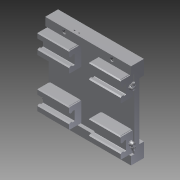
# Autodesk Inventor part: GL20NL-typeExNY Table
Saved by Autodesk Inventor 2011 SP1 (Build 150282100, 282)
## iProperties
Created: 2013-11-12
Part Number: GL20NL-typeExNY Table
Catalog Web Link: www.cadenas.de
Description: Type GL-N-Y - Table2-
Vendor: THK
Document SubType Name: Modeling
Designer: PARTuser1
Manufacturer: THK
Density: 1 g/cm^3
Category: PARTsolutions
Company: THK
Title: GL20NL-typeExNY Table
Author: Cadenas PARTsolutions
PSOL_IDENT_0: {$CADENAS_DATA\23d-libs\thk\actuator\type_gl_n\type_gl_n_f_na_s20.prj},199 {VTYP=3D},{NB=GL20NL-type
PSOL_IDENT_1: ExNY Table},{LINA=GL20NL-typeExNY Table},{NN=Type GL-N-Y - Table2},{DATE=01.03.2011 00:58:01},{GEOMD
PSOL_IDENT_2: ATE=14.11.2007 13:42:00},{VERSION=},{LINEID=60},{LINESUBID=-1},{WBVAR=S}  {NB=GL20NL-typeExNY Table}
PSOL_IDENT_3: ,{LINA=GL20NL-typeExNY Table},{KT=DUMMY},{IDNR=},{MN=GL20N},{TT=L-type},{TL=180},{B=55},{C=100},{D=2
PSOL_IDENT_4: 7},{RF=5.000},{RF2=2.750},{L1=62.000},{L2=66.500},{DS=Ex},{VER=2},{S=N},{LM=SW}
CNS_NN: Type GL-N-Y - Table2
CNS_NB: GL20NL-typeExNY Table
CNS_NBSYN: $MN.$TT.$DS.$S.Y Table
CNS_LINA: GL20NL-typeExNY Table
CNS_MN: GL20N
CNS_TT: L-type
CNS_TL: 180
CNS_B: 55
CNS_C: 100
CNS_D: 27
CNS_RF: 5.000
CNS_RF2: 2.750
CNS_L1: 62.000
CNS_L2: 66.500
CNS_DS: Ex
CNS_VER: 2
CNS_S: N:None
CNS_LM: SW
SUPPLIER: THK
ARTICLENO: GL20NL-typeExNY Table
BOMINFO: GL20NL-typeExNY Table
CREATOR: CADENAS GmbH
Autodesk Inventor part; units mm, degrees
sketch "Sketch_2" plane through (0, 0, 0) normal (1, 0, 0) x (0, 1, 0)
  line L0 (19, 90) -> (19, 73)
  line L1 (19, 73) -> (26, 73)
  line L2 (26, 73) -> (26, -73)
  line L3 (26, -73) -> (19, -73)
  line L4 (19, -73) -> (19, -90)
  line L5 (19, -90) -> (46, -90)
  line L6 (46, -90) -> (46, -60)
  line L7 (46, -60) -> (36.5, -60)
  line L8 (36.5, -60) -> (36.5, 60)
  line L9 (36.5, 60) -> (46, 60)
  line L10 (46, 60) -> (46, 90)
  line L11 (46, 90) -> (19, 90)
  constraints: 24 end point
extrude "Extrusion1" add sketch "Sketch_2" along normal mid plane 180
sketch "Sketch_3" plane through (85, 0, 0) normal (1, 0, 0) x (0, 0, -1)
  line L0 (29.75, 25) -> (29.75, 1.8)
  line L1 (29.75, 1.8) -> (30.5, 1.05)
  line L2 (30.5, 1.05) -> (30.5, 24.6)
  line L3 (30.5, 24.6) -> (31.5, 25.6)
  line L4 (31.5, 25.6) -> (45.55, 25.6)
  line L5 (45.55, 25.6) -> (45.25, 26)
  line L6 (45.25, 26) -> (30.75, 26)
  line L7 (30.75, 26) -> (29.75, 25)
  constraints: 16 end point
extrude "Extrusion2" add sketch "Sketch_3" against normal blind 62
sketch "Sketch_4" plane through (85, 0, 0) normal (1, 0, 0) x (0, 0, -1)
  line L0 (56.45, 25.6) -> (70.5, 25.6)
  line L1 (70.5, 25.6) -> (71.5, 24.6)
  line L2 (71.5, 24.6) -> (71.5, 1.05)
  line L3 (71.5, 1.05) -> (72.25, 1.8)
  line L4 (72.25, 1.8) -> (72.25, 25)
  line L5 (72.25, 25) -> (71.25, 26)
  line L6 (71.25, 26) -> (56.75, 26)
  line L7 (56.75, 26) -> (56.45, 25.6)
  constraints: 16 end point
extrude "Extrusion3" add sketch "Sketch_4" against normal blind 62
sketch "Sketch_5" plane through (87.25, 0, 0) normal (1, 0, 0) x (0, 0, -1)
  line L0 (30.5, 24.6) -> (30.5, 1)
  line L1 (30.5, 1) -> (31.5, 0)
  line L2 (31.5, 0) -> (40.7, 0)
  line L3 (40.7, 0) -> (42.7, 2)
  line L4 (42.7, 2) -> (42.7, 5.5)
  line L5 (42.7, 5.5) -> (40.7, 7.5)
  line L6 (40.7, 7.5) -> (40.7, 10.72)
  line L7 (40.7, 10.72) -> (41.48, 11.5)
  line L8 (41.48, 11.5) -> (60.52, 11.5)
  line L9 (60.52, 11.5) -> (61.3, 10.72)
  line L10 (61.3, 10.72) -> (61.3, 7.5)
  line L11 (61.3, 7.5) -> (59.3, 5.5)
  line L12 (59.3, 5.5) -> (59.3, 2)
  line L13 (59.3, 2) -> (61.3, 0)
  line L14 (61.3, 0) -> (70.5, 0)
  line L15 (70.5, 0) -> (71.5, 1)
  line L16 (71.5, 1) -> (71.5, 24.6)
  line L17 (71.5, 24.6) -> (70.5, 25.6)
  line L18 (70.5, 25.6) -> (31.5, 25.6)
  line L19 (31.5, 25.6) -> (30.5, 24.6)
  constraints: 40 end point
extrude "Extrusion4" add sketch "Sketch_5" against normal blind 66.5
sketch "Sketch_6" plane through (85, 0, 0) normal (1, 0, 0) x (0, 0, -1)
  line L0 (-72.25, 25) -> (-72.25, 1.8)
  line L1 (-72.25, 1.8) -> (-71.5, 1.05)
  line L2 (-71.5, 1.05) -> (-71.5, 24.6)
  line L3 (-71.5, 24.6) -> (-70.5, 25.6)
  line L4 (-70.5, 25.6) -> (-56.45, 25.6)
  line L5 (-56.45, 25.6) -> (-56.75, 26)
  line L6 (-56.75, 26) -> (-71.25, 26)
  line L7 (-71.25, 26) -> (-72.25, 25)
  constraints: 16 end point
extrude "Extrusion5" add sketch "Sketch_6" against normal blind 62
sketch "Sketch_7" plane through (85, 0, 0) normal (1, 0, 0) x (0, 0, -1)
  line L0 (-45.55, 25.6) -> (-31.5, 25.6)
  line L1 (-31.5, 25.6) -> (-30.5, 24.6)
  line L2 (-30.5, 24.6) -> (-30.5, 1.05)
  line L3 (-30.5, 1.05) -> (-29.75, 1.8)
  line L4 (-29.75, 1.8) -> (-29.75, 25)
  line L5 (-29.75, 25) -> (-30.75, 26)
  line L6 (-30.75, 26) -> (-45.25, 26)
  line L7 (-45.25, 26) -> (-45.55, 25.6)
  constraints: 16 end point
extrude "Extrusion6" add sketch "Sketch_7" against normal blind 62
sketch "Sketch_8" plane through (87.25, 0, 0) normal (1, 0, 0) x (0, 0, -1)
  line L0 (-71.5, 24.6) -> (-71.5, 1)
  line L1 (-71.5, 1) -> (-70.5, 0)
  line L2 (-70.5, 0) -> (-61.3, 0)
  line L3 (-61.3, 0) -> (-59.3, 2)
  line L4 (-59.3, 2) -> (-59.3, 5.5)
  line L5 (-59.3, 5.5) -> (-61.3, 7.5)
  line L6 (-61.3, 7.5) -> (-61.3, 10.72)
  line L7 (-61.3, 10.72) -> (-60.52, 11.5)
  line L8 (-60.52, 11.5) -> (-41.48, 11.5)
  line L9 (-41.48, 11.5) -> (-40.7, 10.72)
  line L10 (-40.7, 10.72) -> (-40.7, 7.5)
  line L11 (-40.7, 7.5) -> (-42.7, 5.5)
  line L12 (-42.7, 5.5) -> (-42.7, 2)
  line L13 (-42.7, 2) -> (-40.7, 0)
  line L14 (-40.7, 0) -> (-31.5, 0)
  line L15 (-31.5, 0) -> (-30.5, 1)
  line L16 (-30.5, 1) -> (-30.5, 24.6)
  line L17 (-30.5, 24.6) -> (-31.5, 25.6)
  line L18 (-31.5, 25.6) -> (-70.5, 25.6)
  line L19 (-70.5, 25.6) -> (-71.5, 24.6)
  constraints: 40 end point
extrude "Extrusion7" add sketch "Sketch_8" against normal blind 66.5
sketch "Sketch_9" plane through (-85, 0, 0) normal (1, 0, 0) x (0, 0, -1)
  line L0 (29.75, 25) -> (29.75, 1.8)
  line L1 (29.75, 1.8) -> (30.5, 1.05)
  line L2 (30.5, 1.05) -> (30.5, 24.6)
  line L3 (30.5, 24.6) -> (31.5, 25.6)
  line L4 (31.5, 25.6) -> (45.55, 25.6)
  line L5 (45.55, 25.6) -> (45.25, 26)
  line L6 (45.25, 26) -> (30.75, 26)
  line L7 (30.75, 26) -> (29.75, 25)
  constraints: 16 end point
extrude "Extrusion8" add sketch "Sketch_9" along normal blind 62
sketch "Sketch_10" plane through (-85, 0, 0) normal (1, 0, 0) x (0, 0, -1)
  line L0 (56.45, 25.6) -> (70.5, 25.6)
  line L1 (70.5, 25.6) -> (71.5, 24.6)
  line L2 (71.5, 24.6) -> (71.5, 1.05)
  line L3 (71.5, 1.05) -> (72.25, 1.8)
  line L4 (72.25, 1.8) -> (72.25, 25)
  line L5 (72.25, 25) -> (71.25, 26)
  line L6 (71.25, 26) -> (56.75, 26)
  line L7 (56.75, 26) -> (56.45, 25.6)
  constraints: 16 end point
extrude "Extrusion9" add sketch "Sketch_10" along normal blind 62
sketch "Sketch_11" plane through (-87.25, 0, 0) normal (1, 0, 0) x (0, 0, -1)
  line L0 (30.5, 24.6) -> (30.5, 1)
  line L1 (30.5, 1) -> (31.5, 0)
  line L2 (31.5, 0) -> (40.7, 0)
  line L3 (40.7, 0) -> (42.7, 2)
  line L4 (42.7, 2) -> (42.7, 5.5)
  line L5 (42.7, 5.5) -> (40.7, 7.5)
  line L6 (40.7, 7.5) -> (40.7, 10.72)
  line L7 (40.7, 10.72) -> (41.48, 11.5)
  line L8 (41.48, 11.5) -> (60.52, 11.5)
  line L9 (60.52, 11.5) -> (61.3, 10.72)
  line L10 (61.3, 10.72) -> (61.3, 7.5)
  line L11 (61.3, 7.5) -> (59.3, 5.5)
  line L12 (59.3, 5.5) -> (59.3, 2)
  line L13 (59.3, 2) -> (61.3, 0)
  line L14 (61.3, 0) -> (70.5, 0)
  line L15 (70.5, 0) -> (71.5, 1)
  line L16 (71.5, 1) -> (71.5, 24.6)
  line L17 (71.5, 24.6) -> (70.5, 25.6)
  line L18 (70.5, 25.6) -> (31.5, 25.6)
  line L19 (31.5, 25.6) -> (30.5, 24.6)
  constraints: 40 end point
extrude "Extrusion10" add sketch "Sketch_11" along normal blind 66.5
sketch "Sketch_12" plane through (-85, 0, 0) normal (1, 0, 0) x (0, 0, -1)
  line L0 (-72.25, 25) -> (-72.25, 1.8)
  line L1 (-72.25, 1.8) -> (-71.5, 1.05)
  line L2 (-71.5, 1.05) -> (-71.5, 24.6)
  line L3 (-71.5, 24.6) -> (-70.5, 25.6)
  line L4 (-70.5, 25.6) -> (-56.45, 25.6)
  line L5 (-56.45, 25.6) -> (-56.75, 26)
  line L6 (-56.75, 26) -> (-71.25, 26)
  line L7 (-71.25, 26) -> (-72.25, 25)
  constraints: 16 end point
extrude "Extrusion11" add sketch "Sketch_12" along normal blind 62
sketch "Sketch_13" plane through (-85, 0, 0) normal (1, 0, 0) x (0, 0, -1)
  line L0 (-45.55, 25.6) -> (-31.5, 25.6)
  line L1 (-31.5, 25.6) -> (-30.5, 24.6)
  line L2 (-30.5, 24.6) -> (-30.5, 1.05)
  line L3 (-30.5, 1.05) -> (-29.75, 1.8)
  line L4 (-29.75, 1.8) -> (-29.75, 25)
  line L5 (-29.75, 25) -> (-30.75, 26)
  line L6 (-30.75, 26) -> (-45.25, 26)
  line L7 (-45.25, 26) -> (-45.55, 25.6)
  constraints: 16 end point
extrude "Extrusion12" add sketch "Sketch_13" along normal blind 62
sketch "Sketch_14" plane through (-87.25, 0, 0) normal (1, 0, 0) x (0, 0, -1)
  line L0 (-71.5, 24.6) -> (-71.5, 1)
  line L1 (-71.5, 1) -> (-70.5, 0)
  line L2 (-70.5, 0) -> (-61.3, 0)
  line L3 (-61.3, 0) -> (-59.3, 2)
  line L4 (-59.3, 2) -> (-59.3, 5.5)
  line L5 (-59.3, 5.5) -> (-61.3, 7.5)
  line L6 (-61.3, 7.5) -> (-61.3, 10.72)
  line L7 (-61.3, 10.72) -> (-60.52, 11.5)
  line L8 (-60.52, 11.5) -> (-41.48, 11.5)
  line L9 (-41.48, 11.5) -> (-40.7, 10.72)
  line L10 (-40.7, 10.72) -> (-40.7, 7.5)
  line L11 (-40.7, 7.5) -> (-42.7, 5.5)
  line L12 (-42.7, 5.5) -> (-42.7, 2)
  line L13 (-42.7, 2) -> (-40.7, 0)
  line L14 (-40.7, 0) -> (-31.5, 0)
  line L15 (-31.5, 0) -> (-30.5, 1)
  line L16 (-30.5, 1) -> (-30.5, 24.6)
  line L17 (-30.5, 24.6) -> (-31.5, 25.6)
  line L18 (-31.5, 25.6) -> (-70.5, 25.6)
  line L19 (-70.5, 25.6) -> (-71.5, 24.6)
  constraints: 40 end point
extrude "Extrusion13" add sketch "Sketch_14" along normal blind 66.5
sketch "Sketch14" plane through (-90, 19, -73) normal (0, -1, 0) x (1, 0, 0)
  point P0 (40, -9.5)
hole "Drilling 1" at (-50, 19, -82.5) direction (0, 1, 0) diameter 6.647 depth 27 countersink diameter 8 countersink angle 90 thread size "M8x1.25" class "6H" standard "ISO Metric profile"
sketch "Sketch15" plane through (-90, 19, 90) normal (0, -1, 0) x (1, 0, 0)
  point P0 (40, -7.5)
hole "Drilling 2" at (-50, 19, 82.5) direction (0, 1, 0) diameter 6.647 depth 27 countersink diameter 8 countersink angle 90 thread size "M8x1.25" class "6H" standard "ISO Metric profile"
sketch "Sketch16" plane through (-90, 19, -73) normal (0, -1, 0) x (1, 0, 0)
  point P0 (140, -9.5)
hole "Drilling 3" at (50, 19, -82.5) direction (0, 1, 0) diameter 6.647 depth 27 countersink diameter 8 countersink angle 90 thread size "M8x1.25" class "6H" standard "ISO Metric profile"
sketch "Sketch17" plane through (-90, 19, 90) normal (0, -1, 0) x (1, 0, 0)
  point P0 (140, -7.5)
hole "Drilling 4" at (50, 19, 82.5) direction (0, 1, 0) diameter 6.647 depth 27 countersink diameter 8 countersink angle 90 thread size "M8x1.25" class "6H" standard "ISO Metric profile"
sketch "Sketch_19" plane through (-35, 0, 0) normal (1, 0, 0) x (0, 0, -1)
  line L0 (-84, 25.5) -> (-90, 25.5)
  line L1 (-90, 25.5) -> (-90, 27)
  line L2 (-90, 27) -> (-89.7295, 26.7295)
  line L3 (-89.7295, 26.7295) -> (-84.2705, 26.7295)
  line L4 (-84.2705, 26.7295) -> (-84, 27)
  line L5 (-84, 27) -> (-84, 25.5)
  line L6 (-84, 25.5) -> (-90, 25.5)
  constraints: 14 end point
revolve "Revolution1" cut sketch "Sketch_19" angle 360 about axis through (-35, 25.5, 84) along (0, 0, -1)
thread "Thread1" size "M3x0.5" class "6H" standard "ISO Metric profile" full length
sketch "Sketch_20" plane through (-25, 0, 0) normal (1, 0, 0) x (0, 0, -1)
  line L0 (-84, 25.5) -> (-90, 25.5)
  line L1 (-90, 25.5) -> (-90, 27)
  line L2 (-90, 27) -> (-89.7295, 26.7295)
  line L3 (-89.7295, 26.7295) -> (-84.2705, 26.7295)
  line L4 (-84.2705, 26.7295) -> (-84, 27)
  line L5 (-84, 27) -> (-84, 25.5)
  line L6 (-84, 25.5) -> (-90, 25.5)
  constraints: 14 end point
revolve "Revolution2" cut sketch "Sketch_20" angle 360 about axis through (-25, 25.5, 84) along (0, 0, -1)
thread "Thread2" size "M3x0.5" class "6H" standard "ISO Metric profile" full length
sketch "Sketch_25" plane through (87.25, 0, 0) normal (1, 0, 0) x (0, 0, -1)
  line L0 (47, 22.8094) -> (47, 18.1906)
  line L1 (47, 18.1906) -> (51, 15.8812)
  line L2 (51, 15.8812) -> (55, 18.1906)
  line L3 (55, 18.1906) -> (55, 22.8094)
  line L4 (55, 22.8094) -> (51, 25.1188)
  line L5 (51, 25.1188) -> (47, 22.8094)
  constraints: 12 end point
extrude "Extrusion14" add sketch "Sketch_25" along normal blind 2.14
sketch "Sketch_26" plane through (87.25, 0, 0) normal (1, 0, 0) x (0, 0, -1)
  line L0 (-55, 22.8094) -> (-55, 18.1906)
  line L1 (-55, 18.1906) -> (-51, 15.8812)
  line L2 (-51, 15.8812) -> (-47, 18.1906)
  line L3 (-47, 18.1906) -> (-47, 22.8094)
  line L4 (-47, 22.8094) -> (-51, 25.1188)
  line L5 (-51, 25.1188) -> (-55, 22.8094)
  constraints: 12 end point
extrude "Extrusion15" add sketch "Sketch_26" along normal blind 2.14
sketch "Sketch_27" plane through (-87.25, 0, 0) normal (1, 0, 0) x (0, 0, -1)
  line L0 (47, 22.8094) -> (47, 18.1906)
  line L1 (47, 18.1906) -> (51, 15.8812)
  line L2 (51, 15.8812) -> (55, 18.1906)
  line L3 (55, 18.1906) -> (55, 22.8094)
  line L4 (55, 22.8094) -> (51, 25.1188)
  line L5 (51, 25.1188) -> (47, 22.8094)
  constraints: 12 end point
extrude "Extrusion16" add sketch "Sketch_27" against normal blind 2.14
sketch "Sketch_28" plane through (-87.25, 0, 0) normal (1, 0, 0) x (0, 0, -1)
  line L0 (-55, 22.8094) -> (-55, 18.1906)
  line L1 (-55, 18.1906) -> (-51, 15.8812)
  line L2 (-51, 15.8812) -> (-47, 18.1906)
  line L3 (-47, 18.1906) -> (-47, 22.8094)
  line L4 (-47, 22.8094) -> (-51, 25.1188)
  line L5 (-51, 25.1188) -> (-55, 22.8094)
  constraints: 12 end point
extrude "Extrusion17" add sketch "Sketch_28" against normal blind 2.14
sketch "Sketch_21" plane through (0, 0, -51) normal (0, 0, 1) x (1, 0, 0)
  line L0 (95.79, 20.5) -> (89.39, 20.5)
  line L1 (89.39, 20.5) -> (89.39, 24.5)
  line L2 (89.39, 24.5) -> (92.59, 24.5)
  arc A0 (95.79, 20.5) -> (92.59, 24.5) centre (92.692, 21.3016) ccw
  line L3 (95.79, 20.5) -> (89.39, 20.5)
  constraints: 8 end point, 2 point on circle, 1 centre point
revolve "Revolution3" add sketch "Sketch_21" angle 360 about axis through (95.79, 20.5, -51) along (1, 0, 0)
sketch "Sketch_22" plane through (0, 0, -51) normal (0, 0, 1) x (1, 0, 0)
  line L0 (-89.39, 20.5) -> (-95.79, 20.5)
  arc A0 (-92.59, 24.5) -> (-95.79, 20.5) centre (-92.692, 21.3016) ccw
  line L1 (-92.59, 24.5) -> (-89.39, 24.5)
  line L2 (-89.39, 24.5) -> (-89.39, 20.5)
  line L3 (-89.39, 20.5) -> (-95.79, 20.5)
  constraints: 8 end point, 2 point on circle, 1 centre point
revolve "Revolution4" add sketch "Sketch_22" angle 360 about axis through (-89.39, 20.5, -51) along (1, 0, 0)
sketch "Sketch_23" plane through (0, 0, 51) normal (0, 0, 1) x (1, 0, 0)
  line L0 (95.79, 20.5) -> (89.39, 20.5)
  line L1 (89.39, 20.5) -> (89.39, 24.5)
  line L2 (89.39, 24.5) -> (92.59, 24.5)
  arc A0 (95.79, 20.5) -> (92.59, 24.5) centre (92.692, 21.3016) ccw
  line L3 (95.79, 20.5) -> (89.39, 20.5)
  constraints: 8 end point, 2 point on circle, 1 centre point
revolve "Revolution5" add sketch "Sketch_23" angle 360 about axis through (95.79, 20.5, 51) along (1, 0, 0)
sketch "Sketch_24" plane through (0, 0, 51) normal (0, 0, 1) x (1, 0, 0)
  line L0 (-89.39, 20.5) -> (-95.79, 20.5)
  arc A0 (-92.59, 24.5) -> (-95.79, 20.5) centre (-92.692, 21.3016) ccw
  line L1 (-92.59, 24.5) -> (-89.39, 24.5)
  line L2 (-89.39, 24.5) -> (-89.39, 20.5)
  line L3 (-89.39, 20.5) -> (-95.79, 20.5)
  constraints: 8 end point, 2 point on circle, 1 centre point
revolve "Revolution6" add sketch "Sketch_24" angle 360 about axis through (-89.39, 20.5, 51) along (1, 0, 0)
sketch "Sketch_37" plane through (72.4444, 0, 19.4114) normal (0.9659258, 0, 0.258819) x (0.258819, 0, -0.9659258)
  line L0 (84.25, 20.5) -> (75.75, 20.5)
  line L1 (75.75, 20.5) -> (75.75, 23.5)
  line L2 (75.75, 23.5) -> (77.58, 23.5)
  line L3 (77.58, 23.5) -> (77.78, 24.7)
  line L4 (77.78, 24.7) -> (79.58, 24.7)
  line L5 (79.58, 24.7) -> (79.58, 24)
  line L6 (79.58, 24) -> (81.28, 23.35)
  line L7 (81.28, 23.35) -> (82.02, 23.545)
  line L8 (82.02, 23.545) -> (84.25, 22.65)
  line L9 (84.25, 22.65) -> (84.25, 20.5)
  line L10 (84.25, 20.5) -> (75.75, 20.5)
  constraints: 22 end point
revolve "Revolution7" add sketch "Sketch_37" angle 360 about axis through (94.2499, 20.5, -61.9678) along (0.258819, 0, -0.9659258)
sketch "Sketch_38" plane through (-72.4444, 0, -19.4114) normal (0.9659258, 0, 0.258819) x (0.258819, 0, -0.9659258)
  line L0 (-75.75, 20.5) -> (-84.25, 20.5)
  line L1 (-84.25, 20.5) -> (-84.25, 22.65)
  line L2 (-84.25, 22.65) -> (-82.02, 23.545)
  line L3 (-82.02, 23.545) -> (-81.28, 23.35)
  line L4 (-81.28, 23.35) -> (-79.58, 24)
  line L5 (-79.58, 24) -> (-79.58, 24.7)
  line L6 (-79.58, 24.7) -> (-77.78, 24.7)
  line L7 (-77.78, 24.7) -> (-77.58, 23.5)
  line L8 (-77.58, 23.5) -> (-75.75, 23.5)
  line L9 (-75.75, 23.5) -> (-75.75, 20.5)
  line L10 (-75.75, 20.5) -> (-84.25, 20.5)
  constraints: 22 end point
revolve "Revolution8" add sketch "Sketch_38" angle 360 about axis through (-92.05, 20.5, 53.7575) along (0.258819, 0, -0.9659258)
sketch "Sketch_39" plane through (72.4444, 0, -19.4114) normal (-0.9659258, 0, 0.258819) x (0.258819, 0, 0.9659258)
  line L0 (84.25, 20.5) -> (75.75, 20.5)
  line L1 (75.75, 20.5) -> (75.75, 23.5)
  line L2 (75.75, 23.5) -> (77.58, 23.5)
  line L3 (77.58, 23.5) -> (77.78, 24.7)
  line L4 (77.78, 24.7) -> (79.58, 24.7)
  line L5 (79.58, 24.7) -> (79.58, 24)
  line L6 (79.58, 24) -> (81.28, 23.35)
  line L7 (81.28, 23.35) -> (82.02, 23.545)
  line L8 (82.02, 23.545) -> (84.25, 22.65)
  line L9 (84.25, 22.65) -> (84.25, 20.5)
  line L10 (84.25, 20.5) -> (75.75, 20.5)
  constraints: 22 end point
revolve "Revolution9" add sketch "Sketch_39" angle 360 about axis through (94.2499, 20.5, 61.9678) along (0.258819, 0, 0.9659258)
sketch "Sketch_40" plane through (-72.4444, 0, 19.4114) normal (-0.9659258, 0, 0.258819) x (0.258819, 0, 0.9659258)
  line L0 (-75.75, 20.5) -> (-84.25, 20.5)
  line L1 (-84.25, 20.5) -> (-84.25, 22.65)
  line L2 (-84.25, 22.65) -> (-82.02, 23.545)
  line L3 (-82.02, 23.545) -> (-81.28, 23.35)
  line L4 (-81.28, 23.35) -> (-79.58, 24)
  line L5 (-79.58, 24) -> (-79.58, 24.7)
  line L6 (-79.58, 24.7) -> (-77.78, 24.7)
  line L7 (-77.78, 24.7) -> (-77.58, 23.5)
  line L8 (-77.58, 23.5) -> (-75.75, 23.5)
  line L9 (-75.75, 23.5) -> (-75.75, 20.5)
  line L10 (-75.75, 20.5) -> (-84.25, 20.5)
  constraints: 22 end point
revolve "Revolution10" add sketch "Sketch_40" angle 360 about axis through (-92.05, 20.5, -53.7575) along (0.258819, 0, 0.9659258)
sketch "Sketch_47" plane through (20.0844, 0, -74.9558) normal (-0.258819, 0, 0.9659258) x (0.9659258, 0, 0.258819)
  line L0 (70, 15.5) -> (85, 15.5)
  line L1 (85, 15.5) -> (85, 25.5)
  line L2 (85, 25.5) -> (70, 25.5)
  line L3 (70, 25.5) -> (70, 15.5)
  line L4 (70.9585, 20.5) -> (72.9793, 17)
  line L5 (72.9793, 17) -> (77.0207, 17)
  line L6 (77.0207, 17) -> (79.0415, 20.5)
  line L7 (79.0415, 20.5) -> (77.0207, 24)
  line L8 (77.0207, 24) -> (72.9793, 24)
  line L9 (72.9793, 24) -> (70.9585, 20.5)
  constraints: 20 end point
extrude "Extrusion18" cut sketch "Sketch_47" against normal blind 2
sketch "Sketch_48" plane through (-20.0844, 0, 74.9558) normal (-0.258819, 0, 0.9659258) x (0.9659258, 0, 0.258819)
  line L0 (-85, 15.5) -> (-70, 15.5)
  line L1 (-70, 15.5) -> (-70, 25.5)
  line L2 (-70, 25.5) -> (-85, 25.5)
  line L3 (-85, 25.5) -> (-85, 15.5)
  line L4 (-79.1015, 20.5) -> (-77.0807, 17)
  line L5 (-77.0807, 17) -> (-73.0393, 17)
  line L6 (-73.0393, 17) -> (-71.0185, 20.5)
  line L7 (-71.0185, 20.5) -> (-73.0393, 24)
  line L8 (-73.0393, 24) -> (-77.0807, 24)
  line L9 (-77.0807, 24) -> (-79.1015, 20.5)
  constraints: 20 end point
extrude "Extrusion19" cut sketch "Sketch_48" along normal blind 2
sketch "Sketch_49" plane through (20.0844, 0, 74.9558) normal (0.258819, 0, 0.9659258) x (0.9659258, 0, -0.258819)
  line L0 (70, 15.5) -> (85, 15.5)
  line L1 (85, 15.5) -> (85, 25.5)
  line L2 (85, 25.5) -> (70, 25.5)
  line L3 (70, 25.5) -> (70, 15.5)
  line L4 (70.9585, 20.5) -> (72.9793, 17)
  line L5 (72.9793, 17) -> (77.0207, 17)
  line L6 (77.0207, 17) -> (79.0415, 20.5)
  line L7 (79.0415, 20.5) -> (77.0207, 24)
  line L8 (77.0207, 24) -> (72.9793, 24)
  line L9 (72.9793, 24) -> (70.9585, 20.5)
  constraints: 20 end point
extrude "Extrusion20" cut sketch "Sketch_49" along normal blind 2
sketch "Sketch_50" plane through (-20.0844, 0, -74.9558) normal (0.258819, 0, 0.9659258) x (0.9659258, 0, -0.258819)
  line L0 (-85, 15.5) -> (-70, 15.5)
  line L1 (-70, 15.5) -> (-70, 25.5)
  line L2 (-70, 25.5) -> (-85, 25.5)
  line L3 (-85, 25.5) -> (-85, 15.5)
  line L4 (-79.0415, 20.5) -> (-77.0207, 17)
  line L5 (-77.0207, 17) -> (-72.9793, 17)
  line L6 (-72.9793, 17) -> (-70.9585, 20.5)
  line L7 (-70.9585, 20.5) -> (-72.9793, 24)
  line L8 (-72.9793, 24) -> (-77.0207, 24)
  line L9 (-77.0207, 24) -> (-79.0415, 20.5)
  constraints: 20 end point
extrude "Extrusion21" cut sketch "Sketch_50" against normal blind 2
ref_plane "type_gl_n_t1_XY" through (-90, 0, 0) normal (1, 0, 0) x (0, 0, -1)
ref_plane "type_gl_n_t1_YZ" through (-90, 0, 0) normal (0, 0, -1) x (0, 1, 0)
ref_plane "type_gl_n_t1_ZX" through (-90, 0, 0) normal (0, 1, 0) x (1, 0, 0)
body "Solid1"
